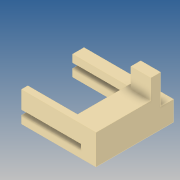
# Autodesk Inventor part: PCB_Holder
Saved by Autodesk Inventor 2019 (Build 230136000, 136)
## iProperties
Created: 2019-02-19
Part Number: PCB_Holder
Material: 일반
Document SubType Name: Modeling
Designer: Jeong Ji Hoon
Density: 1 g/cm^3
Appearance: 기본값
Author: Jeong Ji Hoon
Autodesk Inventor part; units mm, degrees
ref_plane "YZ Plane" through (0, 0, 0) normal (1, 0, 0) x (0, 1, 0)
ref_plane "XZ Plane" through (0, 0, 0) normal (0, 1, 0) x (-1, 0, 0)
ref_plane "XY Plane" through (0, 0, 0) normal (0, 0, 1) x (1, 0, 0)
sketch "스케치1" plane through (0, 0, 0) normal (0, 1, 0) x (-1, 0, 0)
  line L0 (0, 0) -> (0, -15.6)
  line L1 (0, -15.6) -> (18, -15.6)
  line L2 (0, 0) -> (15, 0)
  line L3 (15, 0) -> (15, -1.3)
  line L4 (15, -1.3) -> (5, -1.3)
  line L5 (5, -1.3) -> (5, -5.3)
  line L6 (5, -5.3) -> (4, -5.3)
  line L7 (4, -5.3) -> (4, -9.3)
  line L8 (4, -9.3) -> (5, -9.3)
  line L9 (5, -9.3) -> (5, -13.3)
  line L10 (5, -13.3) -> (18, -13.3)
  line L11 (18, -13.3) -> (18, -15.6)
  line L12 (3, 0) -> (19.1, 0) construction
  line L13 (19.1, 0) -> (19.1, -14.6) construction
  line L14 (19.1, -14.6) -> (3, -14.6) construction
  line L15 (3, -14.6) -> (3, 0) construction
  line L16 (19.1, -7.3) -> (3, -7.3) construction
  dimension "d0" = 15.6
  dimension "d1" = 18
  dimension "d2" = 15
  dimension "d3" = 1.3
  dimension "d4" = 10
  dimension "d5" = 4
  dimension "d6" = 1
  dimension "d7" = 4
  dimension "d8" = 1
  dimension "d9" = 4
  dimension "d10" = 13
  dimension "d18" = 16.1
  dimension "d19" = 14.6
  dimension "d20" = 3
  dimension "d21" = 1
  constraints: 34 end point, 4 horizontal, 4 perpendicular, 3 point on line, 3 vertical, 2 midpoint, 2 parallel
  measures "d0" distance of L0.start L0.end
  measures "d1" distance of L0.end L1.end
  measures "d2" distance of L0.start L2.end
  measures "d3" distance of L2.end L3.end
  measures "d4" distance of L3.end L4.end
  measures "d5" distance of L4.end L5.end
  measures "d6" distance of L5.end L6.end
  measures "d7" distance of L6.end L7.end
  measures "d8" distance of L7.end L8.end
  measures "d9" distance of L8.end L9.end
  measures "d10" distance of L9.end L10.end
  measures "d18" distance of L13.end L14.end
  measures "d19" distance of L12.end L13.end
  measures "d20" distance between parallel lines of L15 L0
  measures "d21" distance between parallel lines of L14 L1
extrude "돌출1" add sketch "스케치1" along normal blind 4
sketch "스케치2" plane through (-15, 0, 0) normal (0, 0, 1) x (1, 0, 0)
  line L0 (-3, 1.5) -> (12, 1.5)
  line L1 (12, 1.5) -> (12, 2.5)
  line L2 (12, 2.5) -> (-3, 2.5)
  line L3 (-3, 2.5) -> (-3, 1.5)
  line L4 (15, 0) -> (15, 4) projected
  line L5 (0, 0) -> (0, 4) projected
  line L6 (0, 0) -> (15, 0) projected
  line L7 (-3, 0) -> (-3, 4) projected
  dimension "d13" = 1
  dimension "d14" = 3
  dimension "d15" = 1.5
  constraints: 8 end point, 2 parallel, 1 horizontal, 1 perpendicular, 1 point on line
  measures "d13" distance of L1.end L0.end
  measures "d14" distance between parallel lines of L1 L4
  measures "d15" distance between parallel lines of L6 L0
extrude "돌출2" cut sketch "스케치2" against normal blind 14.6
sketch "스케치3" plane through (0, 4, 0) normal (0, 1, 0) x (1, 0, 0)
  line L0 (0, 0) -> (0, 15.6) projected
  line L1 (0, 15.6) -> (-18, 15.6) projected
  line L2 (0, 0) -> (-4, 0)
  line L3 (-4, 0) -> (-4, 13)
  line L4 (-4, 13) -> (0, 13)
  line L5 (0, 13) -> (0, 0)
  line L6 (-15, 0) -> (0, 0) projected
  point P0 (-3, 0)
  dimension "d22" = 4
  dimension "d23" = 13
  constraints: 8 end point, 2 parallel, 2 point on line, 1 horizontal, 1 perpendicular
  measures "d22" distance of L3.end L4.end
  measures "d23" distance of L2.end L3.end
extrude "돌출3" add sketch "스케치3" along normal blind 2
sketch "스케치4" plane through (0, 6, 0) normal (0, 1, 0) x (1, 0, 0)
  line L0 (0, 0) -> (0, 15.6) projected
  line L1 (-4, 13) -> (0, 13)
  line L2 (0, 13) -> (0, 11)
  line L3 (0, 11) -> (-4, 11)
  line L4 (-4, 11) -> (-4, 13)
  line L5 (0, 0) -> (0, 13) projected
  line L6 (0, 13) -> (-4, 13) projected
  line L7 (-4, 13) -> (-4, 0) projected
  line L8 (-4, 0) -> (0, 0) projected
  dimension "d26" = 2
  constraints: 8 end point, 2 parallel, 1 horizontal, 1 perpendicular, 1 point on line
  measures "d26" distance of L1.end L2.end
extrude "돌출4" add sketch "스케치4" along normal blind 4 contours L3 L4 L1 L0
sketch "스케치5" plane through (0, 4, 0) normal (0, 1, 0) x (1, 0, 0)
  line L0 (-4, 0) -> (-4, 5.3) projected
  line L1 (-4, 5.3) -> (-5, 5.3) projected
  line L2 (-5, 5.3) -> (-5, 1.3) projected
  line L3 (-5, 1.3) -> (-15, 1.3) projected
  line L4 (-15, 1.3) -> (-15, 0) projected
  line L5 (-15, 0) -> (-4, 0) projected
  line L6 (-4, 9.3) -> (-4, 13) projected
  line L7 (-4, 13) -> (0, 13) projected
  line L8 (0, 13) -> (0, 15.6) projected
  line L9 (0, 15.6) -> (-18, 15.6) projected
  line L10 (-18, 15.6) -> (-18, 13.3) projected
  line L11 (-18, 13.3) -> (-5, 13.3) projected
  line L12 (-5, 13.3) -> (-5, 9.3) projected
  line L13 (-5, 9.3) -> (-4, 9.3) projected
  line L14 (-4, 0) -> (-5, 0)
  line L15 (-5, 0) -> (-5, 13)
  line L16 (-5, 13) -> (-4, 13)
  line L17 (-4, 13) -> (-4, 0)
  point P0 (0, 0)
  dimension "d31" = 13
  constraints: 8 end point, 2 parallel, 1 horizontal, 1 perpendicular, 1 point on line
  measures "d31" distance of L14.end L15.end
extrude "돌출5" add sketch "스케치5" along normal blind 2 contours L5 L15 L2 L1 L0 | L1 L15 L13 L17 | L5 L4 L3 L15 | L13 L12 L16 L6
